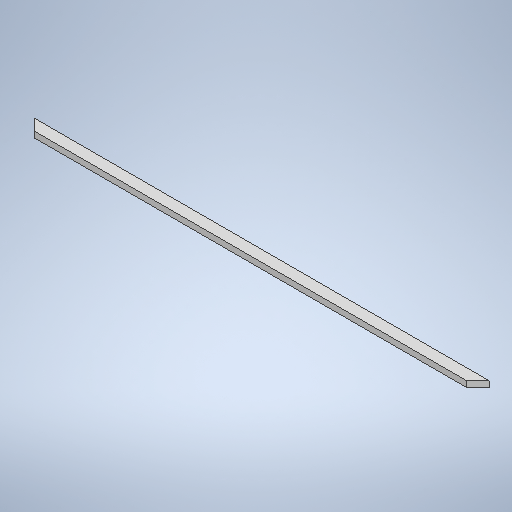
# Autodesk Inventor part: DitchtungRahmen
Saved by Autodesk Inventor 2025.1 (Build 291241000, 241)
## iProperties
Created: 2024-08-07
Part Number: DitchtungRahmen
Material: Generisch
Document SubType Name: Modeling
Designer: ffogue
Density: 1 g/cm^3
Appearance: Vorgabe
Author: ffogue
Autodesk Inventor part; units mm, degrees
ref_plane "YZ Plane" through (0, 0, 0) normal (1, 0, 0) x (0, 1, 0)
ref_plane "XZ Plane" through (0, 0, 0) normal (0, 1, 0) x (-1, 0, 0)
ref_plane "XY Plane" through (0, 0, 0) normal (0, 0, 1) x (1, 0, 0)
sketch "Sketch1" plane through (0, 0, 0) normal (0, 0, 1) x (1, 0, 0)
  line L0 (0, 0) -> (770, 0)
  line L1 (770, 0) -> (770, 19)
  line L2 (770, 19) -> (0, 19)
  line L3 (0, 19) -> (0, 0)
  dimension "d0" = 19
  dimension "d1" = 770
  constraints: 8 end point, 2 parallel, 1 horizontal, 1 perpendicular
  measures "d0" distance between parallel lines of L2 L0
  measures "d1" distance of L1.end L2.end
extrude "Extrusion1" add sketch "Sketch1" along normal mid plane 10
sketch "Sketch2" plane through (0, 0, 5) normal (0, 0, 1) x (1, 0, 0)
  line L0 (770, 0) -> (770, 19) projected
  line L1 (770, 19) -> (0, 19) projected
  line L2 (0, 19) -> (0, 0) projected
  line L3 (0, 0) -> (770, 0) projected
  line L4 (0, 19) -> (19, 0)
  line L5 (770, 19) -> (751, 0)
  line L6 (0, 0) -> (770, 0) projected
  line L7 (385, 0) -> (385, 48.3121) construction
  dimension "d8" = 45
  constraints: 6 end point, 2 point on line, 1 midpoint, 1 symmetric about line, 1 vertical
  measures "d8" angle of L4 L2
extrude "Extrusion2" cut sketch "Sketch2" against normal blind 10 contours L3 L5 L0 | L4 L3 L2
equation "\"d1\" = DichBrei"
equation "\"DichBrei\" = 770"
body "Solid1"
